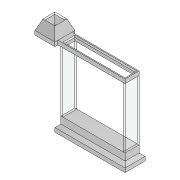
# Autodesk Inventor part: Box
Saved by Autodesk Inventor 2021 (Build 250183000, 183)
## iProperties
Created: 2021-04-01
Part Number: Box
Material: Generic
Document SubType Name: Modeling
Designer: Tran Duc Viet
Mass: 2891.33 g
Surface Area: 3098.98 cm^2
Volume: 2891.33 cm^3
Density: 1 g/cm^3
Appearance: Default
Author: Tran Duc Viet
Autodesk Inventor part; units mm, degrees
sketch "Sketch1" plane through (0, 0, 0) normal (0, 1, 0) x (-1, 0, 0)
  line L0 (150, 25) -> (-150, 25)
  line L1 (-150, 25) -> (-150, -25)
  line L2 (-150, -25) -> (150, -25)
  line L3 (150, -25) -> (150, 25)
  line L4 (150, 25) -> (-150, -25) construction
  line L5 (-150, 25) -> (150, -25) construction
  line L6 (160, 35) -> (-160, 35)
  line L7 (-160, 35) -> (-160, -35)
  line L8 (-160, -35) -> (160, -35)
  line L9 (160, -35) -> (160, 35)
  line L10 (160, 35) -> (-160, -35) construction
  line L11 (-160, 35) -> (160, -35) construction
  point P0 (0, 0)
  dimension "d0" = 300
  dimension "d1" = 50
  dimension "d2" = 320
  dimension "d3" = 70
  constraints: 24 end point, 4 midpoint, 4 parallel, 2 horizontal, 2 perpendicular
  measures "d0" distance of L2.end L1.end
  measures "d1" distance of L1.end L0.end
  measures "d2" distance of L8.end L7.end
  measures "d3" distance of L8.end L6.start
extrude "Extrusion1" add sketch "Sketch1" along normal blind 320
ref_plane "Work Plane1" through (0, 300, 0) normal (0, 1, 0) x (1, 0, 0)
sketch "Sketch2" plane through (0, 0, 0) normal (0, -1, 0) x (1, 0, 0)
  line L0 (160, 35) -> (160, -35) projected
  line L1 (-160, -35) -> (160, -35)
  line L2 (160, -35) -> (160, 35)
  line L3 (160, 35) -> (-160, 35)
  line L4 (-160, 35) -> (-160, -35)
  line L5 (-160, -35) -> (160, 35) construction
  line L6 (160, -35) -> (-160, 35) construction
  point P0 (0, 0)
  constraints: 12 end point, 2 midpoint, 2 parallel, 1 horizontal, 1 perpendicular
extrude "Extrusion2" add sketch "Sketch2" along normal blind 50
sketch "Sketch3" plane through (0, -50, 0) normal (0, -1, 0) x (1, 0, 0)
  line L0 (-175, -50) -> (175, -50)
  line L1 (175, -50) -> (175, 50)
  line L2 (175, 50) -> (-175, 50)
  line L3 (-175, 50) -> (-175, -50)
  line L4 (-175, -50) -> (175, 50) construction
  line L5 (175, -50) -> (-175, 50) construction
  point P0 (0, 0)
  dimension "d9" = 350
  dimension "d10" = 100
  constraints: 12 end point, 2 midpoint, 2 parallel, 1 horizontal, 1 perpendicular
  measures "d9" distance of L2.end L1.end
  measures "d10" distance of L1.end L0.end
extrude "Extrusion3" add sketch "Sketch3" along normal blind 20
chamfer "Chamfer1" distance 15 angle 45 4 edges at (0, -50, 35) (-160, -50, 0) (0, -50, -35) (160, -50, 0)
chamfer "Chamfer2" distance 5 angle 45 4 edges at (0, 320, -25) (-150, 320, 0) (0, 320, 25) (150, 320, 0)
split body "Split1" result two bodies by plane through (0, 300, 0) normal (0, 1, 0) first body at (50, 300.5, 31.6667)
ref_plane "Work Plane2" through (0, 0, 0) normal (0, -1, 0) x (1, 0, 0)
split body "Split2" result two bodies by plane through (0, 0, 0) normal (0, -1, 0) bodies 3 first body at (58.3333, -69.5, -16.6667)
sketch "Sketch4" plane through (-160, 300, 35) normal (0, 0, 1) x (1, 0, 0)
  line L0 (10, -300) -> (10, 0) projected
  line L1 (310, -300) -> (310, 0) projected
  line L2 (10, 0) -> (310, 0)
  line L3 (310, 0) -> (310, -300)
  line L4 (310, -300) -> (10, -300)
  line L5 (10, -300) -> (10, 0)
  point P0 (160, -300)
  constraints: 8 end point, 2 parallel, 1 horizontal, 1 perpendicular
extrude "Extrusion4" cut sketch "Sketch4" against normal through all bodies 5
sketch "Sketch5" plane through (0, 320, 0) normal (0, 1, 0) x (1, 0, 0)
  line L0 (-175, -50) -> (-175, 50) projected
  line L1 (-175, 50) -> (-275, 50)
  line L2 (-275, 50) -> (-275, -50)
  line L3 (-275, -50) -> (-175, -50)
  line L4 (-175, -50) -> (-175, 50)
  line L5 (-160, 35) -> (160, 35) projected
  line L6 (-160, 35) -> (-175, 35)
  line L7 (-175, 35) -> (-175, -35)
  line L8 (-175, -35) -> (-160, -35)
  line L9 (-160, -35) -> (-160, 35)
  point P0 (0, 0)
  dimension "d22" = 100
  dimension "d23" = 100
  dimension "d24" = 15
  dimension "d25" = 70
  constraints: 16 end point, 4 parallel, 2 horizontal, 2 perpendicular
  measures "d22" distance of L3.end L2.end
  measures "d23" distance of L2.end L1.end
  measures "d24" distance of L8.end L7.end
  measures "d25" distance of L7.end L6.end
extrude "Extrusion5" add sketch "Sketch5" against normal blind 20 bodies 2
ref_plane "Work Plane3" through (0, 370, 0) normal (0, 1, 0) x (1, 0, 0)
sketch "Sketch7" plane through (0, 370, 0) normal (0, 1, 0) x (1, 0, 0)
  line L0 (-255, 30) -> (-195, 30)
  line L1 (-195, 30) -> (-195, -30)
  line L2 (-195, -30) -> (-255, -30)
  line L3 (-255, -30) -> (-255, 30)
  line L4 (-175, 50) -> (-275, 50) projected
  line L5 (-275, 50) -> (-275, -50) projected
  point P0 (0, 0)
  dimension "d33" = 60
  dimension "d34" = 60
  dimension "d35" = 20
  dimension "d36" = 20
  constraints: 8 end point, 2 parallel, 1 horizontal, 1 perpendicular
  measures "d33" distance of L1.end L2.end
  measures "d34" distance of L0.end L1.end
  measures "d35" distance between parallel lines of L4 L0
  measures "d36" distance between parallel lines of L5 L3
sketch "Sketch8" plane through (0, 320, 0) normal (0, 1, 0) x (1, 0, 0)
  line L0 (-275, 50) -> (-275, -50) projected
  line L1 (-175, -50) -> (-275, -50) projected
  line L2 (-275, 50) -> (-175, 50)
  line L3 (-175, 50) -> (-175, -50)
  line L4 (-175, -50) -> (-275, -50)
  line L5 (-275, -50) -> (-275, 50)
  point P0 (0, 0)
  constraints: 8 end point, 2 parallel, 1 horizontal, 1 perpendicular
loft "Loft1" add profiles "Sketch8", "Sketch7" bodies 2
sketch "Sketch9" plane through (-255, 370, 30) normal (0, 1, 0) x (1, 0, 0)
  line L0 (5, 55) -> (55, 55)
  line L1 (55, 55) -> (55, 5)
  line L2 (55, 5) -> (5, 5)
  line L3 (5, 5) -> (5, 55)
  line L4 (60, 60) -> (0, 60) projected
  line L5 (0, 60) -> (0, 0) projected
  point P0 (255, 30)
  dimension "d41" = 50
  dimension "d42" = 50
  dimension "d43" = 5
  dimension "d44" = 5
  constraints: 8 end point, 2 parallel, 1 horizontal, 1 perpendicular
  measures "d41" distance of L1.end L2.end
  measures "d42" distance of L0.end L1.end
  measures "d43" distance between parallel lines of L4 L0
  measures "d44" distance between parallel lines of L5 L3
extrude "Extrusion6" cut sketch "Sketch9" against normal blind 50 bodies 2
chamfer "Chamfer3" distance 5 angle 45 4 edges at (-225, 370, -25) (-200, 370, 0) (-225, 370, 25) (-250, 370, 0)
equation "\"d4\" = d2"
